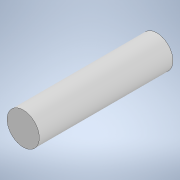
# Autodesk Inventor part: CilindroHidraulico_1
Saved by Autodesk Inventor 2021 (Build 250183000, 183)
## iProperties
Created: 2021-07-12
Part Number: CilindroHidraulico_1
Material: Generic
Document SubType Name: Modeling
Designer: Nelson
Density: 1 g/cm^3
Appearance: Default
Author: Nelson
Autodesk Inventor part; units mm, degrees
ref_plane "YZ Plane" through (0, 0, 0) normal (1, 0, 0) x (0, 1, 0)
ref_plane "XZ Plane" through (0, 0, 0) normal (0, 1, 0) x (-1, 0, 0)
ref_plane "XY Plane" through (0, 0, 0) normal (0, 0, 1) x (1, 0, 0)
sketch "Sketch2" plane through (0, 0, 0) normal (1, 0, 0) x (0, 1, 0)
  line L0 (0, 0) -> (80, 0)
  line L1 (80, -662) -> (0, -662)
  line L2 (0, -662) -> (0, 0)
  line L3 (0, 0) -> (80, 0)
  line L4 (80, 0) -> (80, -80)
  line L5 (80, -80) -> (10, -80)
  line L6 (80, -662) -> (80, -582)
  line L7 (80, -582) -> (10, -582)
  line L8 (10, -80) -> (10, -582)
  line L9 (80, -80) -> (80, -131) construction
  line L10 (80, -131) -> (152.4165, -131) construction
  line L11 (0, -662) -> (0, -792) construction
  line L12 (0, -792) -> (216.7213, -792) construction
  line L13 (80, -582) -> (80, -531)
  line L14 (80, -531) -> (152.4165, -531)
  dimension "d4" = 80
  dimension "d7" = 662
  dimension "d8" = 80
  dimension "d9" = 80
  dimension "d10" = 70
  dimension "d11" = 80
  dimension "d12" = 70
  dimension "d17" = 51
  dimension "d18" = 130
  dimension "d19" = 51
  constraints: 30 end point, 4 horizontal, 4 vertical, 3 perpendicular, 2 parallel, 1 collinear
  measures "d4" distance of L1.start L1.end
  measures "d7" distance of L1.end L0.start
  measures "d8" distance of L0.start L0.end
  measures "d9" distance of L0.end L4.end
  measures "d10" distance of L4.end L5.end
  measures "d11" distance of L1.start L6.end
  measures "d12" distance of L6.end L7.end
  measures "d17" distance of L4.end L9.end
  measures "d18" distance of L1.end L11.end
  measures "d19" distance of L6.end L13.end
revolve "Revolution1" add sketch "Sketch2" angle 360 about axis through (0, 80, 0) along (0, 0, -1)
sketch "Sketch3" plane through (0, 80, -662) normal (0, 0, -1) x (-1, 0, 0)
  circle A0 centre (0, 0) radius 44.5
  point P0 (0, -80)
  dimension "d14" = 89
  constraints: 1 centre point
  measures "d14" diameter of A0
extrude "Extrusion2" cut sketch "Sketch3" against normal blind 400
equation "\"d4\" = d8"
equation "\"d11\" = d9"
equation "\"d12\" = d10"
body "Solid2"
